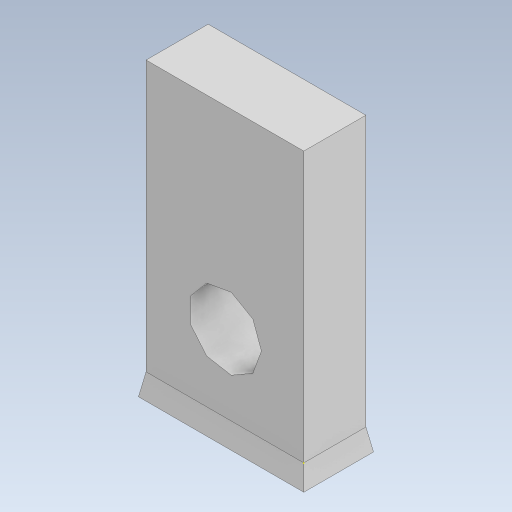
# Autodesk Inventor part: Support Hole
Saved by Autodesk Inventor 2023 (Build 270158000, 158)
## iProperties
Created: 2022-09-14
Part Number: Support Hole
Material: Generic
Document SubType Name: Modeling
Designer: Dave
Density: 1 g/cm^3
Appearance: Default
Author: Dave
Autodesk Inventor part; units mm, degrees
ref_plane "YZ Plane" through (0, 0, 0) normal (1, 0, 0) x (0, 1, 0)
ref_plane "XZ Plane" through (0, 0, 0) normal (0, 1, 0) x (-1, 0, 0)
ref_plane "XY Plane" through (0, 0, 0) normal (0, 0, 1) x (1, 0, 0)
sketch "Sketch1" plane through (0, 0, 0) normal (0, 1, 0) x (-1, 0, 0)
  point P0 (0, 0)
sketch "Sketch2" plane through (0, 0, 0) normal (0, 1, 0) x (-1, 0, 0)
  line L0 (0, 0) -> (14.6, 0)
  line L1 (14.6, 0) -> (14.6, -5.75)
  line L2 (14.6, -5.75) -> (0, -5.75)
  line L3 (0, -5.75) -> (0, 0)
  dimension "d0" = 14.6
  dimension "d1" = 5.75
  constraints: 8 end point, 2 parallel, 1 horizontal, 1 perpendicular
  measures "d0" distance of L1.end L2.end
  measures "d1" distance of L0.end L1.end
extrude "Extrusion1" add sketch "Sketch2" along normal blind 25 and the other way blind 2 draft 10
sketch "Sketch3" plane through (-14.6, 0, 0) normal (0, 0, 1) x (1, 0, 0)
  line L0 (0, 25) -> (14.6, 25) projected
  point P0 (14.6, 0)
  point P1 (7.3, 7)
  point P2 (7.3, 25)
  dimension "d6" = 18
  constraints: 1 midpoint, 1 vertical alignment
  measures "d6" distance from line of L0 point (7.3, 7)
hole "Hole1" at (-7.3, 7, 0) direction (0, 0, -1) diameter 6.7564 depth 12.7 tip angle 118 clearance for "Flat Head Machine Screw (82)" size "1/4" standard "Ansi Unified Screw Threads"
body "Solid1"
